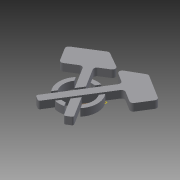
# Autodesk Inventor part: Boilermake_PCBMechanicalOverlay
Saved by Autodesk Inventor 2014 (Build 180170000, 170)
## iProperties
Created: 2014-09-13
Part Number: Boilermake_PCBMechanicalOverlay
Material: Generic
Document SubType Name: Modeling
Designer: Leeroy
Density: 1 g/cm^3
Appearance: Default
Author: Leeroy
Autodesk Inventor part; units mm, degrees
ref_plane "YZ Plane" through (0, 0, 0) normal (1, 0, 0) x (0, 1, 0)
ref_plane "XZ Plane" through (0, 0, 0) normal (0, 1, 0) x (-1, 0, 0)
ref_plane "XY Plane" through (0, 0, 0) normal (0, 0, 1) x (1, 0, 0)
ref_plane "Work Plane3" through (0, 0, 1) normal (0, 0, 1) x (1, 0, 0)
sketch "Sketch4" plane through (0, 0, 1) normal (0, 0, 1) x (1, 0, 0)
  line L0 (-26.3961, -42.3953) -> (15.4675, 24.6005) projected
  arc A0 (20.9794, 25.873) -> (15.4675, 24.6005) centre (18.8597, 22.4808) ccw projected
  line L1 (20.9794, 25.873) -> (34.5482, 17.3943) projected
  arc A1 (34.5482, 17.3943) -> (40.0601, 18.6668) centre (36.6679, 20.7865) ccw projected
  line L2 (40.0601, 18.6668) -> (50.6584, 35.6278) projected
  arc A2 (50.6584, 35.6278) -> (49.3859, 41.1397) centre (47.2663, 37.7475) ccw projected
  line L3 (49.3859, 41.1397) -> (18.3431, 60.5374) projected
  arc A3 (18.3431, 60.5374) -> (14.2342, 60.6155) centre (16.2234, 57.1452) ccw projected
  line L4 (14.2342, 60.6155) -> (-5.4504, 49.3323) projected
  arc A4 (-5.4504, 49.3323) -> (-5.5809, 42.4698) centre (-3.4612, 45.8619) ccw projected
  line L5 (-5.5809, 42.4698) -> (5.7146, 35.4116) projected
  arc A5 (6.9871, 29.8997) -> (5.7146, 35.4116) centre (3.5949, 32.0194) ccw projected
  line L6 (6.9871, 29.8997) -> (-34.8766, -37.0961) projected
  arc A6 (-34.8766, -37.0961) -> (-34.2403, -39.852) centre (-33.1805, -38.1559) ccw projected
  line L7 (-34.2403, -39.852) -> (-29.152, -43.0315) projected
  arc A7 (-29.152, -43.0315) -> (-26.3961, -42.3953) centre (-28.0922, -41.3354) ccw projected
  line L8 (-55.041, 17.3943) -> (-41.4722, 25.873) projected
  arc A8 (-60.5529, 18.6668) -> (-55.041, 17.3943) centre (-57.1607, 20.7865) ccw projected
  line L9 (-71.1513, 35.6278) -> (-60.5529, 18.6668) projected
  arc A9 (-69.8787, 41.1397) -> (-71.1513, 35.6278) centre (-67.7591, 37.7475) ccw projected
  line L10 (-38.8359, 60.5374) -> (-69.8787, 41.1397) projected
  line L11 (-15.0424, 49.3323) -> (-34.727, 60.6155) projected
  arc A10 (-34.727, 60.6155) -> (-38.8359, 60.5374) centre (-36.7162, 57.1452) ccw projected
  arc A11 (-14.9119, 42.4698) -> (-15.0424, 49.3323) centre (-17.0316, 45.8619) ccw projected
  line L12 (-26.2074, 35.4116) -> (-14.9119, 42.4698) projected
  arc A12 (-26.2074, 35.4116) -> (-27.4799, 29.8997) centre (-24.0877, 32.0194) ccw projected
  arc A13 (-35.9604, 24.6005) -> (-41.4722, 25.873) centre (-39.3526, 22.4808) ccw projected
  line L13 (-35.9604, 24.6005) -> (-17.9111, -4.2844) projected
  line L14 (-12.0152, 5.151) -> (-27.4799, 29.8997) projected
  line L15 (-17.9111, -4.2844) -> (-12.0152, 5.151) projected
  arc A14 (-7.3172, 12.6693) -> (-13.1756, 12.6693) centre (-10.2464, -7.115) ccw projected
  line L16 (-16.5715, 18.1039) -> (-13.1756, 12.6693) projected
  arc A15 (-3.9213, 18.1039) -> (-16.5715, 18.1039) centre (-10.2464, -7.115) ccw projected
  line L17 (-7.3172, 12.6693) -> (-3.9213, 18.1039) projected
  line L18 (-26.3961, -42.3953) -> (15.4675, 24.6005) projected
  arc A16 (20.9794, 25.873) -> (15.4675, 24.6005) centre (18.8597, 22.4808) ccw projected
  line L19 (20.9794, 25.873) -> (34.5482, 17.3943) projected
  arc A17 (34.5482, 17.3943) -> (40.0601, 18.6668) centre (36.6679, 20.7865) ccw projected
  line L20 (40.0601, 18.6668) -> (50.6584, 35.6278) projected
  arc A18 (50.6584, 35.6278) -> (49.3859, 41.1397) centre (47.2663, 37.7475) ccw projected
  line L21 (49.3859, 41.1397) -> (18.3431, 60.5374) projected
  arc A19 (18.3431, 60.5374) -> (14.2342, 60.6155) centre (16.2234, 57.1452) ccw projected
  line L22 (14.2342, 60.6155) -> (-5.4504, 49.3323) projected
  arc A20 (-5.4504, 49.3323) -> (-5.5809, 42.4698) centre (-3.4612, 45.8619) ccw projected
  line L23 (-5.5809, 42.4698) -> (5.7146, 35.4116) projected
  arc A21 (6.9871, 29.8997) -> (5.7146, 35.4116) centre (3.5949, 32.0194) ccw projected
  line L24 (6.9871, 29.8997) -> (-34.8766, -37.0961) projected
  arc A22 (-34.8766, -37.0961) -> (-34.2403, -39.852) centre (-33.1805, -38.1559) ccw projected
  line L25 (-34.2403, -39.852) -> (-29.152, -43.0315) projected
  arc A23 (-29.152, -43.0315) -> (-26.3961, -42.3953) centre (-28.0922, -41.3354) ccw projected
  line L26 (-12.0152, 5.151) -> (-27.4799, 29.8997) projected
  arc A24 (-26.2074, 35.4116) -> (-27.4799, 29.8997) centre (-24.0877, 32.0194) ccw projected
  line L27 (-26.2074, 35.4116) -> (-14.9119, 42.4698) projected
  arc A25 (-14.9119, 42.4698) -> (-15.0424, 49.3323) centre (-17.0316, 45.8619) ccw projected
  line L28 (-15.0424, 49.3323) -> (-34.727, 60.6155) projected
  arc A26 (-34.727, 60.6155) -> (-38.8359, 60.5374) centre (-36.7162, 57.1452) ccw projected
  line L29 (-38.8359, 60.5374) -> (-69.8787, 41.1397) projected
  arc A27 (-69.8787, 41.1397) -> (-71.1513, 35.6278) centre (-67.7591, 37.7475) ccw projected
  line L30 (-71.1513, 35.6278) -> (-60.5529, 18.6668) projected
  arc A28 (-60.5529, 18.6668) -> (-55.041, 17.3943) centre (-57.1607, 20.7865) ccw projected
  line L31 (-55.041, 17.3943) -> (-41.4722, 25.873) projected
  arc A29 (-35.9604, 24.6005) -> (-41.4722, 25.873) centre (-39.3526, 22.4808) ccw projected
  line L32 (-35.9604, 24.6005) -> (-17.9111, -4.2844) projected
  line L33 (-17.9111, -4.2844) -> (-12.0152, 5.151) projected
  line L34 (9.6475, 9.6252) -> (6.2516, 4.1906) projected
  arc A30 (6.2516, -18.4206) -> (6.2516, 4.1906) centre (-10.2464, -7.115) ccw projected
  line L35 (6.2516, -18.4206) -> (9.6475, -23.8552) projected
  arc A31 (9.6475, -23.8552) -> (9.6475, 9.6252) centre (-10.2464, -7.115) ccw projected
  line L36 (-30.1403, -23.8552) -> (-26.7444, -18.4206) projected
  arc A32 (-26.7444, 4.1906) -> (-26.7444, -18.4206) centre (-10.2464, -7.115) ccw projected
  line L37 (-26.7444, 4.1906) -> (-30.1403, 9.6252) projected
  arc A33 (-30.1403, 9.6252) -> (-30.1403, -23.8552) centre (-10.2464, -7.115) ccw projected
  line L38 (-13.1756, -26.8993) -> (-16.5715, -32.3339) projected
  arc A34 (-16.5715, -32.3339) -> (-3.9213, -32.3339) centre (-10.2464, -7.115) ccw projected
  line L39 (-3.9213, -32.3339) -> (-7.3172, -26.8993) projected
  arc A35 (-13.1756, -26.8993) -> (-7.3172, -26.8993) centre (-10.2464, -7.115) ccw projected
  line L40 (14.3837, -37.0961) -> (-2.5817, -9.9456) projected
  line L41 (-2.5817, -9.9456) -> (-8.4776, -19.381) projected
  line L42 (-8.4776, -19.381) -> (5.9033, -42.3953) projected
  arc A36 (5.9033, -42.3953) -> (8.6592, -43.0315) centre (7.5994, -41.3354) ccw projected
  line L43 (8.6592, -43.0315) -> (13.7475, -39.852) projected
  arc A37 (13.7475, -39.852) -> (14.3837, -37.0961) centre (12.6876, -38.1559) ccw projected
  point P0 (0, 0)
extrude "Extrusion5" add sketch "Sketch4" along normal blind 10
body "Solid2"
